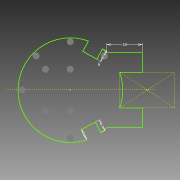
# Autodesk Inventor part: Pi Cam Holder
Saved by Autodesk Inventor 2014 (Build 180170000, 170)
## iProperties
Created: 2016-01-01
Part Number: Pi Cam Holder
Material: Generisch
Document SubType Name: Modeling
Designer: nrk
Density: 1 g/cm^3
Appearance: Vorgabe
Author: nrk
Autodesk Inventor part; units mm, degrees
ref_plane "YZ Plane" through (0, 0, 0) normal (1, 0, 0) x (0, 1, 0)
ref_plane "XZ Plane" through (0, 0, 0) normal (0, 1, 0) x (-1, 0, 0)
ref_plane "XY Plane" through (0, 0, 0) normal (0, 0, 1) x (1, 0, 0)
sketch "Teller" plane through (0, 0, 0) normal (0, 1, 0) x (-1, 0, 0)
  line L0 (-16.2935, -20.8991) -> (-13.3783, -15.6549)
  line L1 (-13.3783, -15.6549) -> (-6.2348, -19.626)
  line L2 (-6.2348, -19.626) -> (-9.15, -24.8702)
  line L3 (-8.2927, 25.1691) -> (-5.5764, 19.8191)
  line L4 (-5.5764, 19.8191) -> (-12.7097, 16.1974)
  line L5 (-12.7097, 16.1974) -> (-15.426, 21.5474)
  arc A0 (-9.15, -24.8702) -> (-8.2927, 25.1691) centre (0, 0) ccw
  line L6 (33, 0) -> (-43, 0) construction
  line L7 (-25, -9) -> (-53, -9) construction
  line L8 (-53, -9) -> (-53, 9) construction
  line L9 (-53, 9) -> (-25, 9) construction
  line L10 (-25, 9) -> (-25, -9) construction
  line L11 (-25, -9) -> (-53, 9) construction
  line L12 (-53, -9) -> (-25, 9) construction
  line L13 (-36.473, -9) -> (-24.9249, -9)
  line L14 (-18.473, -19) -> (-36.473, -19)
  line L15 (-36.473, -19) -> (-36.473, -9)
  line L16 (-36.473, 9) -> (-24.9249, 9)
  line L17 (-18.473, 19) -> (-36.473, 19)
  line L18 (-36.473, 19) -> (-36.473, 9)
  arc A1 (-15.426, 21.5474) -> (-18.473, 19) centre (0, 0) ccw
  arc A2 (-24.9249, 9) -> (-24.9249, -9) centre (0, 0) ccw
  arc A3 (-18.473, -19) -> (-16.2935, -20.8991) centre (0, 0) ccw
  point P0 (-39, 0)
  dimension "d55" = 6
  dimension "d118" = 6
  dimension "d119" = 6
  dimension "d123" = 18
  constraints: 38 end point, 8 point on circle, 5 parallel, 4 centre point, 4 symmetric about line, 3 horizontal, 3 perpendicular, 2 midpoint, 2 point on line
  measures "d55" distance of L3.start L4.start
  measures "d118" distance of L1.start L0.start
  measures "d119" distance of L5.end L4.end
  measures "d123" distance of L14.start L14.end
sketch "Dicke Stifte Außen" plane through (0, 0, 0) normal (0, 1, 0) x (-1, 0, 0)
  line L0 (-29.5209, 0) -> (35.6564, 0) construction
  line L1 (0, -38.3382) -> (0, 35) construction
  circle A0 centre (0, -24.4) radius 1.75
  circle A1 centre (0, 0) radius 26.5 construction
  circle A2 centre (17.2534, -17.2534) radius 1.75
  circle A3 centre (24.4, 0) radius 1.75
  circle A4 centre (17.2534, 17.2534) radius 1.75
  circle A5 centre (0, 24.4) radius 1.75
  circle A6 centre (-17.2534, 17.2534) radius 1.75
  circle A7 centre (-24.4, 0) radius 1.75
  circle A8 centre (-17.2534, -17.2534) radius 1.75
  dimension "d83" = 3.5
  dimension "d84" = 53
  dimension "d87" = 360
  constraints: 9 centre point, 4 end point, 1 coincident, 1 horizontal, 1 perpendicular, 1 point on line, 17 other
  measures "d83" diameter of A0
  measures "d84" diameter of A1
sketch "Dünne Stifte Außen" plane through (0, 0, 0) normal (0, 1, 0) x (-1, 0, 0)
  circle A0 centre (0, -24.4) radius 1
  circle A1 centre (0, 0) radius 26.5 construction
  circle A2 centre (0, 0) radius 26.5 construction
  circle A3 centre (17.2534, -17.2534) radius 1
  circle A4 centre (24.4, 0) radius 1
  circle A5 centre (17.2534, 17.2534) radius 1
  circle A6 centre (0, 24.4) radius 1
  circle A7 centre (-17.2534, 17.2534) radius 1
  circle A8 centre (-24.4, 0) radius 1
  circle A9 centre (-17.2534, -17.2534) radius 1
  dimension "d90" = 2
  dimension "d91" = 53
  dimension "d92" = 53
  dimension "d95" = 360
  constraints: 10 centre point, 2 coincident, 17 other
  measures "d90" diameter of A0
  measures "d91" diameter of A1
  measures "d92" diameter of A2
sketch "Dicke Stifte Vorn" plane through (0, 0, 0) normal (0, 1, 0) x (-1, 0, 0)
  circle A0 centre (0, 10.5) radius 1.75
  line L0 (-29.5209, 0) -> (35.6564, 0) construction
  circle A1 centre (0, -10.5) radius 1.75
  point P0 (0, 0)
  dimension "d97" = 3.5
  constraints: 2 centre point, 2 end point, 1 horizontal, 1 symmetric about line, 1 other
  measures "d97" diameter of A0
sketch "Dicke Stifte Hinten" plane through (0, 0, 0) normal (0, 1, 0) x (-1, 0, 0)
  circle A0 centre (12.5, -10.5) radius 1.75
  line L0 (-29.5209, 0) -> (35.6564, 0) construction
  circle A1 centre (12.5, 10.5) radius 1.75
  point P0 (0, 0)
  dimension "d99" = 3.5
  constraints: 2 centre point, 2 end point, 1 horizontal
  measures "d99" diameter of A0
sketch "Dünne Stifte Vorn" plane through (0, 0, 0) normal (0, 1, 0) x (-1, 0, 0)
  circle A0 centre (0, 10.5) radius 1
  line L0 (-29.5209, 0) -> (35.6564, 0) construction
  circle A1 centre (0, -10.5) radius 1
  point P0 (0, 0)
  dimension "d100" = 2
  constraints: 2 centre point, 2 end point, 1 horizontal, 1 symmetric about line, 1 other
  measures "d100" diameter of A0
sketch "Dünne Stifte Hinten" plane through (0, 0, 0) normal (0, 1, 0) x (-1, 0, 0)
  circle A0 centre (12.5, -10.5) radius 1
  line L0 (-29.5209, 0) -> (35.6564, 0) construction
  circle A1 centre (12.5, 10.5) radius 1
  point P0 (0, 0)
  dimension "d101" = 2
  constraints: 2 centre point, 2 end point, 1 horizontal
  measures "d101" diameter of A0
extrude "Extrusion13" add sketch "Dicke Stifte Außen" along normal blind 8 contours A0 | A2 | A3 | A4 | A5 | A6 | A8
extrude "Extrusion14" add sketch "Dicke Stifte Vorn" along normal blind 4
extrude "Extrusion15" add sketch "Dicke Stifte Hinten" along normal blind 4
extrude "Extrusion16" add sketch "Dünne Stifte Außen" along normal blind 10 contours A0 | A3 | A4 | A5 | A6 | A7 | A9
extrude "Extrusion17" add sketch "Dünne Stifte Vorn" along normal blind 10
extrude "Extrusion18" add sketch "Dünne Stifte Hinten" along normal blind 6
